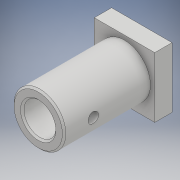
# Autodesk Inventor part: Инж_граф_1
Saved by Autodesk Inventor 2019.3 (Build 233278000, 278)
## iProperties
Created: 2020-03-23
Part Number: Инж_граф_1
Material: Типовые
Document SubType Name: Modeling
Designer: Diana
Density: 1 g/cm^3
Appearance: По умолчанию
Author: Diana
Autodesk Inventor part; units mm, degrees
ref_plane "YZ Plane" through (0, 0, 0) normal (1, 0, 0) x (0, 1, 0)
ref_plane "XZ Plane" through (0, 0, 0) normal (0, 1, 0) x (-1, 0, 0)
ref_plane "XY Plane" through (0, 0, 0) normal (0, 0, 1) x (1, 0, 0)
sketch "Эскиз1" plane through (0, 0, 0) normal (0, 0, 1) x (1, 0, 0)
  line L0 (17.5, -17.5) -> (-17.5, -17.5)
  line L1 (-17.5, -17.5) -> (-17.5, 17.5)
  line L2 (-17.5, 17.5) -> (17.5, 17.5)
  line L3 (17.5, 17.5) -> (17.5, -17.5)
  line L4 (17.5, -17.5) -> (-17.5, 17.5) construction
  line L5 (-17.5, -17.5) -> (17.5, 17.5) construction
  point P0 (0, 0)
  dimension "d0" = 35
  dimension "d1" = 35
  constraints: 12 end point, 2 midpoint, 2 parallel, 1 horizontal, 1 perpendicular
  measures "d0" distance of L0.start L0.end
  measures "d1" distance of L0.start L2.end
extrude "Выдавливание1" add sketch "Эскиз1" against normal blind 10
sketch "Эскиз2" plane through (0, 0, 0) normal (0, 0, 1) x (1, 0, 0)
  circle A0 centre (0, 0) radius 15
  dimension "d4" = 30
  constraints: 1 centre point, 1 coincident
  measures "d4" diameter of A0
extrude "Выдавливание2" add sketch "Эскиз2" along normal blind 50
sketch "Эскиз3" plane through (0, 0, 50) normal (0, 0, 1) x (1, 0, 0)
  point P0 (0, 0)
  point P1 (0, 0)
  constraints: 1 coincident
hole "Отверстие1" at (0, 0, 50) direction (0, 0, -1) diameter 18.5 depth 31 tip angle 120
sketch "Эскиз4" plane through (0, 0, 0) normal (1, 0, 0) x (0, 1, 0)
  circle A0 centre (0, 33) radius 3
  line L0 (0, -22) -> (0, 62) projected
  line L1 (17.5, 0) -> (-17.5, 0) projected
  line L2 (15, 50) -> (-15, 50) projected
  point P0 (0, 0)
  dimension "d14" = 6
  dimension "d15" = 17
  constraints: 1 centre point, 1 point on line
  measures "d14" diameter of A0
  measures "d15" distance from line of L2 A0.centre
extrude "Выдавливание3" cut sketch "Эскиз4" along normal mid plane 50
chamfer "Фаска1" distance 1 angle 45 2 edges at (-15, 0, 50) (0, 9.25, 50)
